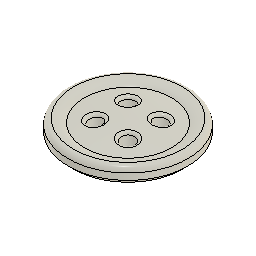
Pants Button v1 (Autodesk Fusion 360 design; units mm, degrees)
Autodesk Fusion 360 part; units mm, degrees
sketch "Sketch1" plane through (0, 0, 0) normal (0, 0, 1) x (1, 0, 0)
  circle A0 centre (0, 0) radius 11
  dimension "d1" = 22
  constraint coincident A0.centre origin
  measures "d1" diameter of A0
extrude "Extrude1" add sketch "Sketch1" along normal blind 3.175
fillet "Fillet1" radius 1 1 edges at (-10.2556, -3.9778, 3.175)
chamfer "Chamfer1" distance 1 angle 45 1 edges at (-10.2556, -3.9778, 0)
sketch "Sketch2" plane through (0, 0, 0) normal (0, 1, 0) x (1, 0, 0)
  arc A0 (0, -3.175) -> (8.0104, -2.425) centre (0, 39.978) ccw
  line L0 (10, -3.175) -> (-10, -3.175)
  line L1 (-11, -2.175) -> (11, -2.175)
  arc A1 (8.0104, -2.425) -> (10, -3.175) centre (10, -0.1611) ccw
  line L2 (0, -3.175) -> (10, -3.175)
  dimension "d7" = 0.75
  dimension "d8" = 3
  constraint tangent A0 L0
  constraint midpoint A0.start L0
  constraint tangent L0 A1
  constraint coincident L0.start A1.end
  constraint midpoint L0 A0.start
  measures "d7" distance of L2 A0.end
  measures "d8" distance of L1.end A0.end
revolve "Revolve1" cut sketch "Sketch2" angle 360 about axis through (0, 0, 1.75) along (0, 0, 1)
sketch "Sketch3" plane through (0, 0, 0) normal (0, 0, 1) x (1, 0, 0)
  line L0 (3, -3) -> (-3, -3) construction
  line L1 (-3, -3) -> (-3, 3) construction
  line L2 (-3, 3) -> (3, 3) construction
  line L3 (3, 3) -> (3, -3) construction
  line L4 (3, -3) -> (-3, 3) construction
  line L5 (-3, -3) -> (3, 3) construction
  circle A0 centre (-3, 3) radius 1.25
  circle A1 centre (3, 3) radius 1.25
  circle A2 centre (3, -3) radius 1.25
  circle A3 centre (-3, -3) radius 1.25
  dimension "d9" = 6
  dimension "d10" = 2.5
  constraint perpendicular L0 L1
  constraint parallel L0 L2
  constraint parallel L1 L3
  constraint horizontal L0
  constraint coincident L4 origin
  constraint coincident L5 origin
  constraint equal L2 L3
  constraint coincident L1.end L2.start
  constraint coincident L2.end L3.start
  constraint coincident L0.start L3.end
  constraint coincident L0.end L1.start
  constraint equal A0 A1
  constraint equal A0 A3
  constraint equal A0 A2
  measures "d9" distance of L1.end L2.end
  measures "d10" diameter of A0
extrude "Extrude2" cut sketch "Sketch3" along normal through all and the other way through all
fillet "Fillet2" radius 0.5 4 edges at (-4.25, 3, 2.8603) (1.75, 3, 3.035) (1.75, -3, 3.035) (-4.25, -3, 2.8603)
chamfer "Chamfer2" distance 0.5 angle 45 4 edges at (-4.1654, -3.452, 0) (1.8346, -3.452, 0) (1.8346, 2.548, 0) (-4.1654, 2.548, 0)
